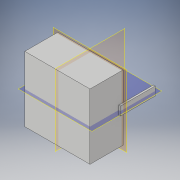
# Autodesk Inventor part: Assembly Mount Mount
Saved by Autodesk Inventor 2019 (Build 230136000, 136)
## iProperties
Created: 2021-02-18
Part Number: Assembly Mount Mount
Material: Generic
Document SubType Name: Modeling
Designer: Eric
Density: 1 g/cm^3
Appearance: Default
Author: Eric
Autodesk Inventor part; units mm, degrees
ref_plane "YZ Plane" through (0, 0, 0) normal (1, 0, 0) x (0, 1, 0)
ref_plane "XZ Plane" through (0, 0, 0) normal (0, 1, 0) x (-1, 0, 0)
ref_plane "XY Plane" through (0, 0, 0) normal (0, 0, 1) x (1, 0, 0)
sketch "Sketch1" plane through (0, 0, 0) normal (0, 0, 1) x (1, 0, 0)
  line L0 (0, 0) -> (75, 0)
  line L1 (75, 0) -> (75, -75)
  line L2 (75, -75) -> (0, -75)
  line L3 (0, -75) -> (0, 0)
  dimension "d0" = 75
  dimension "d1" = 75
  constraints: 8 end point, 2 horizontal, 2 vertical
  measures "d0" distance of L1.end L2.end
  measures "d1" distance of L0.end L1.end
extrude "Extrusion1" add sketch "Sketch1" along normal blind 38
sketch "Sketch2" plane through (75, -75, 0) normal (1, 0, 0) x (0, 0, -1)
  line L0 (0, 75) -> (0, 0) projected
  line L1 (0, 75) -> (-38, 75) projected
  line L2 (0, 0) -> (-38, 0) projected
  line L3 (35, 32.5) -> (-5, 32.5)
  line L4 (-5, 32.5) -> (-5, 42.5)
  line L5 (-5, 42.5) -> (35, 42.5)
  line L6 (35, 42.5) -> (35, 32.5)
  dimension "d4" = 40
  dimension "d5" = 10
  dimension "d6" = 5
  dimension "d7" = 32.5
  dimension "d8" = 32.5
  constraints: 8 end point, 4 parallel
  measures "d4" distance of L4.end L5.end
  measures "d5" distance of L3.end L4.end
  measures "d6" distance between parallel lines of L0 L4
  measures "d7" distance between parallel lines of L2 L3
  measures "d8" distance between parallel lines of L1 L5
extrude "Extrusion2" add sketch "Sketch2" along normal blind 2 separate body
ref_plane "Work Plane1" through (38.5, -75, 0) normal (1, 0, 0) x (0, 0, -1)
ref_plane "Work Plane2" through (0, -37.5, 0) normal (0, -1, 0) x (1, 0, 0)
ref_plane "Work Plane3" through (0, 0, 1.5) normal (0, 0, 1) x (1, 0, 0)
equation "\"d7\" = d8"
body "Solid1"
body "Solid2"
